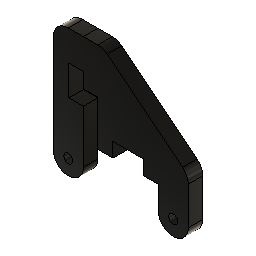
CameraHolderSide v2 (Autodesk Fusion 360 design; units mm, degrees)
Autodesk Fusion 360 part; units mm, degrees
sketch "Sketch1" plane through (0, 0, 0) normal (0, 1, 0) x (1, 0, 0)
  line L0 (-4.8, 0) -> (-4.8, -10)
  line L1 (0, 0) -> (0, -15)
  line L2 (0, -15) -> (-4.8, -15)
  line L3 (0, 0) -> (-4.8, 0) construction
  line L4 (-4.8, 0) -> (-4.8, 7.5)
  line L5 (0, -30) -> (-4.8, -30)
  line L6 (0, -15) -> (0, -30) construction
  line L7 (-4.8, -15) -> (-4.8, -30) construction
  line L8 (-4.8, -30) -> (-9.8, -30)
  line L9 (-14.8, 7.5) -> (-14.8, -25)
  arc A0 (-9.8, -30) -> (-14.8, -25) centre (-9.8, -25) ccw construction
  arc A1 (-14.8, -25) -> (-9.8, -30) centre (-9.8, -25) ccw
  arc A2 (-14.8, 7.5) -> (-4.8, 7.5) centre (-9.8, 7.5) ccw construction
  arc A3 (-4.8, 7.5) -> (-14.8, 7.5) centre (-9.8, 7.5) ccw
  circle A4 centre (-9.8, 7.5) radius 1.5
  line L10 (0, 0) -> (5, 0)
  line L11 (5, 0) -> (5, -4.8)
  line L12 (5, -4.8) -> (15, -4.8)
  line L13 (15, -4.8) -> (15, 0)
  line L14 (15, 0) -> (20, 0)
  line L15 (20, 0) -> (20, 7.5)
  line L16 (30, 7.5) -> (30, -5)
  line L17 (3.1235, -28.9043) -> (28.1235, -8.9043)
  arc A5 (3.1235, -28.9043) -> (0, -30) centre (0, -25) ccw construction
  arc A6 (0, -30) -> (3.1235, -28.9043) centre (0, -25) ccw
  arc A7 (30, -5) -> (28.1235, -8.9043) centre (25, -5) ccw construction
  arc A8 (28.1235, -8.9043) -> (30, -5) centre (25, -5) ccw
  arc A9 (20, 7.5) -> (30, 7.5) centre (25, 7.5) ccw construction
  arc A10 (30, 7.5) -> (20, 7.5) centre (25, 7.5) ccw
  circle A11 centre (25, 7.5) radius 1.5
  line L18 (-4.8, -10) -> (-9.6, -10)
  line L19 (-9.6, -10) -> (-9.6, -20)
  line L20 (-9.6, -20) -> (-4.8, -20)
  line L21 (-4.8, -20) -> (-4.8, -15)
  line L22 (-9.8, 7.5) -> (-9.8, -25) construction
  line L23 (-4.8, 7.5) -> (20, 7.5) construction
  dimension "d1" = 15
  dimension "d3" = 4.8
  dimension "d4" = 7.5
  dimension "d5" = 4.8
  dimension "d6" = 15
  dimension "d7" = 10
  dimension "d8" = 10
  dimension "d9" = 3
  dimension "d10" = 5
  dimension "d11" = 4.8
  dimension "d12" = 10
  dimension "d13" = 4.8
  dimension "d14" = 5
  dimension "d16" = 10
  dimension "d17" = 10
  dimension "d18" = 5
  dimension "d19" = 5
  dimension "d20" = 5
  dimension "d21" = 3
  dimension "d22" = 4.8
  dimension "d23" = 10
  dimension "d24" = 5
  constraint vertical L0
  constraint coincident L1.start L3.start
  constraint vertical L1
  constraint perpendicular L0 L2
  constraint perpendicular L0 L3
  constraint perpendicular L3 L4
  constraint parallel L2 L5
  constraint perpendicular L5 L6
  constraint tangent L7 A0
  constraint tangent L8 A0
  constraint tangent L4 A2
  constraint tangent L9 A0
  constraint vertical L9
  constraint concentric A0 A1
  constraint concentric A2 A3
  constraint concentric A3 A4
  constraint collinear L5 L8
  constraint perpendicular L1 L10
  constraint perpendicular L10 L11
  constraint perpendicular L11 L12
  constraint perpendicular L12 L13
  constraint perpendicular L13 L14
  constraint perpendicular L14 L15
  constraint tangent L15 A9
  constraint coincident L6 A5.centre
  constraint tangent L16 A7
  constraint tangent L17 A7
  constraint tangent L17 A5
  constraint concentric A5 A6
  constraint concentric A7 A8
  constraint concentric A9 A10
  constraint tangent L16 A9
  constraint concentric A10 A11
  constraint perpendicular L0 L18
  constraint perpendicular L18 L19
  constraint coincident L7 L20.end
  constraint perpendicular L7 L20
  constraint perpendicular L2 L21
  constraint coincident A2.centre A3.centre
  constraint coincident A0.centre A1.centre
  constraint perpendicular L3 L22
  constraint perpendicular L15 L23
  measures "d1" distance of L0.start L2.end
  measures "d3" distance of L2.end L1.end
  measures "d4" distance of L0.start L4.end
  measures "d5" distance of L5.start L5.end
  measures "d6" distance of L2 L5
  measures "d7" diameter of A0
  measures "d8" diameter of A2
  measures "d9" diameter of A4
  measures "d10" distance of L1.start L10.end
  measures "d11" distance of L10.end L11.end
  measures "d12" distance of L11.end L12.end
  measures "d13" distance of L12.end L13.end
  measures "d14" distance of L13.end L14.end
  measures "d16" diameter of A9
  measures "d17" diameter of A7
  measures "d18" distance of L14 A7.centre
  measures "d19" radius of A5
  measures "d20" distance of L15 A7.centre
  measures "d21" diameter of A11
  measures "d22" distance of L0.end L18.end
  measures "d23" distance of L18.end L19.end
  measures "d24" distance of L2 L18
extrude "Extrude1" add sketch "Sketch1" along normal blind 4.8
